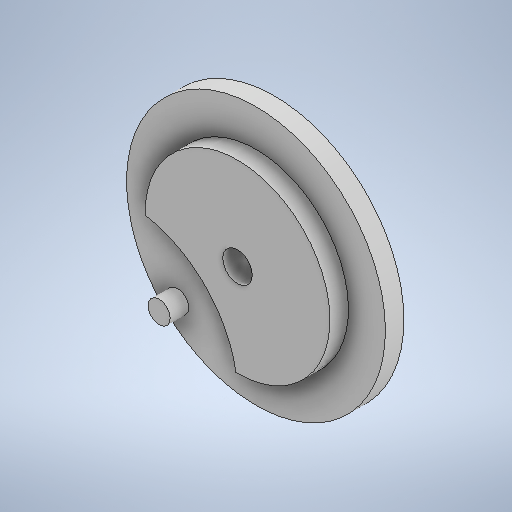
# Autodesk Inventor part: Geneva_driver
Saved by Autodesk Inventor 2025.2 (Build 292293000, 293)
## iProperties
Created: 2025-01-23
Part Number: Geneva_driver
Material: Generic
Document SubType Name: Modeling
Designer: yash3
Density: 1 g/cm^3
Appearance: Default
Author: yash3
Autodesk Inventor part; units mm, degrees
ref_plane "YZ Plane" through (0, 0, 0) normal (1, 0, 0) x (0, 1, 0)
ref_plane "XZ Plane" through (0, 0, 0) normal (0, 1, 0) x (-1, 0, 0)
ref_plane "XY Plane" through (0, 0, 0) normal (0, 0, 1) x (1, 0, 0)
sketch "Sketch1" plane through (0, 0, 0) normal (0, 0, 1) x (1, 0, 0)
  line L0 (0, 0) -> (30, 0) construction
  line L1 (30, 0) -> (30, 30) construction
  line L2 (30, 30) -> (0, 30) construction
  line L3 (0, 11.9722) -> (0, 0) construction
  circle A0 centre (0, 0) radius 30 construction
  circle A1 centre (30, 30) radius 30 construction
  circle A2 centre (30, 30) radius 35
  arc A3 (29.5798, 5.0035) -> (5.0035, 29.5798) centre (30, 30) ccw
  arc A4 (29.5798, 5.0035) -> (5.0035, 29.5798) centre (0, 0) ccw
  line L4 (30, 30) -> (0, 0) construction
  circle A5 centre (30, 30) radius 4
  circle A6 centre (8.7868, 8.7868) radius 3
  dimension "d3" = 60
  dimension "d4" = 70
  dimension "d0" = 30
  dimension "d1" = 30
  dimension "d2" = 60
  dimension "d5" = 50
  dimension "d6" = 8
  dimension "d7" = 6
  constraints: 10 end point, 6 coincident, 6 point on circle, 5 centre point, 2 parallel, 1 horizontal, 1 perpendicular, 1 point on line, 6 other
  measures "d0" distance of L2.end L1.end
  measures "d1" distance of L1.end L0.end
  measures "d2" diameter of A0
  measures "d5" diameter of A3
  measures "d6" diameter of A5
  measures "d7" diameter of A6
extrude "Extrusion1" add sketch "Sketch1" along normal blind 5 contours A4 A3 | A6
extrude "Extrusion2" add sketch "Sketch1" against normal blind 5 contours A2 | A4 A3 | A6
body "Solid1"
